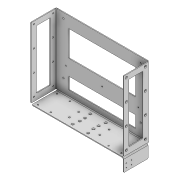
# Autodesk Inventor part: Display_Mount_A
Saved by Autodesk Inventor 2020 (Build 240168000, 168)
## iProperties
Created: 2021-12-05
Part Number: Display_Mount_A
Material: 一般
Document SubType Name: Sheet Metal
Designer: ken113
Density: 1 g/cm^3
Sheet Metal Rule: Default_mm
Appearance: 既定
Flat Pattern Width: 55.1572 cm
Flat Pattern Length: 37.0786 cm
Flat Pattern Area: 2045.15 cm^2
Sheet Metal Width: 551.572 mm
Sheet Metal Length: 370.786 mm
Sheet Metal Area: 204514.969 mm^2
Author: ken113
Autodesk Inventor part; units mm, degrees
ref_plane "YZ Plane" through (0, 0, 0) normal (1, 0, 0) x (0, 1, 0)
ref_plane "XZ Plane" through (0, 0, 0) normal (0, 1, 0) x (-1, 0, 0)
ref_plane "XY Plane" through (0, 0, 0) normal (0, 0, 1) x (1, 0, 0)
sketch "スケッチ1" plane through (0, 0, 0) normal (0, 0, 1) x (1, 0, 0)
  line L0 (175, -135) -> (-175, -135)
  line L1 (-175, -135) -> (-175, 135)
  line L2 (-175, 135) -> (175, 135)
  line L3 (175, 135) -> (175, -135)
  line L4 (175, -135) -> (-175, 135) construction
  line L5 (-175, -135) -> (175, 135) construction
  point P0 (0, 0)
  dimension "d0" = 270
  dimension "d1" = 350
  measures "d0" distance of L0.end L1.end
  measures "d1" distance of L1.end L2.end
extrude "プレート1" add sketch "スケッチ1" along normal blind 3
sketch "スケッチ2" plane through (175, -138, 6) normal (0, -1, 0) x (1, 0, 0)
  line L0 (-350, 0) -> (0, 0)
  line L1 (0, 0) -> (0, 94)
  line L2 (0, 94) -> (-350, 94)
  line L3 (-350, 94) -> (-350, 0)
  constraints: 6 end point, 1 horizontal, 1 perpendicular, 1 vertical
edge flange "フランジ1" height 100 angle 90 thickness 3 bend radius 3 thickness toward (0, -1, 0) relief straight relief width 3 relief depth 1.5 edges at (0, -135, 3) wall of the first edge with corners at (-175, -138, 6) (175, -138, 6) (175, -138, 100) (-175, -138, 100)
bend "曲げ1"
corner "コーナー1"
sketch "スケッチ3" plane through (0, 0, 3) normal (0, 0, 1) x (1, 0, 0)
  line L0 (150, -85) -> (-150, -85)
  line L1 (-150, -85) -> (-150, 115)
  line L2 (-150, 115) -> (150, 115)
  line L3 (150, 115) -> (150, -85)
  line L4 (150, -85) -> (-150, 115) construction
  line L5 (-150, -85) -> (150, 115) construction
  line L6 (175, -135) -> (-175, -135) projected
  point P0 (0, 0)
  point P1 (0, 15)
  dimension "d13" = 300
  dimension "d14" = 200
  dimension "d15" = 50
  constraints: 12 end point, 2 midpoint, 2 parallel, 1 horizontal, 1 perpendicular
  measures "d13" distance of L0.start L0.end
  measures "d14" distance of L0.end L1.end
  measures "d15" distance between parallel lines of L0 L6
hole "穴1" at (-150, 115, 3) at (-150, -85, 3) at (150, -85, 3) at (150, 115, 3) direction (0, 0, -1) diameter 6.2 depth 3 tip angle 118
sketch "スケッチ4" plane through (0, 0, 3) normal (0, 0, 1) x (1, 0, 0)
  line L0 (130, -8.8) -> (-130, -8.8)
  line L1 (-130, -8.8) -> (-130, 91.2)
  line L2 (-130, 91.2) -> (130, 91.2)
  line L3 (130, 91.2) -> (130, -8.8)
  line L4 (130, -8.8) -> (-130, 91.2) construction
  line L5 (-130, -8.8) -> (130, 91.2) construction
  circle A0 centre (-150, 115) radius 3.1 projected
  point P0 (0, 0)
  point P1 (0, 41.2)
  point P2 (0, 41.2)
  dimension "d23" = 100
  dimension "d24" = 23.8
  dimension "d25" = 260
  constraints: 12 end point, 3 midpoint, 2 parallel, 1 horizontal, 1 perpendicular, 1 vertical alignment
  measures "d23" distance of L2.end L0.start
  measures "d24" distance from line of L2 A0.centre
  measures "d25" distance of L1.end L2.end
extrude "押し出し1" cut sketch "スケッチ4" against normal through all contours L0 L1 L2 L3
fillet "フィレット1" radius 2 4 edges at (130, -8.8, 1.5) (130, 91.2, 1.5) (-130, 91.2, 1.5) (-130, -8.8, 1.5)
sketch "スケッチ5" plane through (-175, -138, 100) normal (0, 1, 0) x (1, 0, 0)
  line L0 (350, 94) -> (0, 94) projected
  line L1 (0, 0) -> (0, 94) projected
  line L2 (0, 0) -> (350, 0) projected
  line L3 (350, 0) -> (350, 94) projected
  line L4 (145, 13) -> (205, 13)
  line L5 (205, 13) -> (205, 81)
  line L6 (205, 81) -> (145, 81)
  line L7 (145, 81) -> (145, 13)
  line L8 (145, 13) -> (205, 81) construction
  line L9 (205, 13) -> (145, 81) construction
  line L10 (148.5, 37) -> (201.5, 37)
  line L11 (201.5, 37) -> (201.5, 57)
  line L12 (201.5, 57) -> (148.5, 57)
  line L13 (148.5, 57) -> (148.5, 37)
  line L14 (148.5, 37) -> (201.5, 57) construction
  line L15 (201.5, 37) -> (148.5, 57) construction
  point P0 (175, 100)
  point P1 (175, 47)
  point P2 (175, 0)
  point P3 (175, 47)
  point P4 (0, 47)
  point P5 (175, 47)
  dimension "d29" = 60
  dimension "d30" = 68
  dimension "d31" = 53
  dimension "d32" = 20
  constraints: 24 end point, 8 midpoint, 4 parallel, 2 horizontal, 2 perpendicular, 1 horizontal alignment, 1 vertical alignment
  measures "d29" distance of L6.end L5.end
  measures "d30" distance of L5.end L4.end
  measures "d31" distance of L12.end L11.end
  measures "d32" distance of L11.end L10.end
hole "穴2" at (-30, -138, 19) at (-26.5, -138, 43) at (-26.5, -138, 63) at (26.5, -138, 63) at (26.5, -138, 43) at (30, -138, 19) at (30, -138, 87) at (-30, -138, 87) direction (0, -1, 0) diameter 5.3 depth 3 tip angle 118 countersink diameter 10 countersink angle 90
sketch "スケッチ6" plane through (178, 135, 6) normal (1, 0, 0) x (0, 1, 0)
  line L0 (-270, 0) -> (0, 0)
  line L1 (0, 0) -> (0, 94)
  line L2 (0, 94) -> (-270, 94)
  line L3 (-270, 94) -> (-270, 0)
  constraints: 6 end point, 1 horizontal, 1 perpendicular, 1 vertical
edge flange "フランジ2" height 100 angle 90 thickness 3 bend radius 3 thickness toward (1, 0, 0) relief straight relief width 3 relief depth 1.5 corner gap 3 corner form 0 edges at (175, 0, 3) (-175, 0, 3) wall of the first edge with corners at (178, -135, 6) (178, 135, 6) (178, 135, 100) (178, -135, 100)
bend "曲げ2"
corner "コーナー2"
fillet "フィレット2" radius 2 5 edges at (-179.5, 135, 100) (-179.5, -135, 100) (-175, -139.5, 100) (179.5, -135, 100) (179.5, 135, 100)
sketch "スケッチ7" plane through (181, -135, 6) normal (1, 0, 0) x (0, 0, -1)
  arc A0 (-94, 268) -> (-92, 270) centre (-92, 268) ccw projected
  line L0 (-94, 2) -> (-94, 268) projected
  arc A1 (-92, 0) -> (-94, 2) centre (-92, 2) ccw projected
  line L1 (0, 0) -> (-92, 0) projected
  line L2 (0, 0) -> (0, 270) projected
  line L3 (-92, 270) -> (0, 270)
  line L4 (-10, 260) -> (-10, 16)
  line L5 (-10, 16) -> (-84, 16)
  line L6 (-84, 16) -> (-84, 260)
  line L7 (-84, 260) -> (-10, 260)
  line L8 (-84, 97.3333) -> (-10, 97.3333)
  line L9 (-10, 97.3333) -> (-10, 178.6667)
  line L10 (-10, 178.6667) -> (-84, 178.6667)
  line L11 (-84, 178.6667) -> (-84, 97.3333)
  point P0 (6, 135)
  dimension "d51" = 10
  dimension "d52" = 244
  dimension "d53" = 81.3333
  dimension "d54" = 81.3333
  dimension "d75" = 10
  dimension "d76" = 16
  dimension "d77" = 10
  constraints: 18 end point, 2 centre point, 2 parallel, 2 perpendicular, 2 point on line, 1 horizontal
  measures "d51" distance between parallel lines of L2 L4
  measures "d52" distance of L5.end L6.end
  measures "d53" distance between parallel lines of L7 L10
  measures "d54" distance between parallel lines of L10 L8
  measures "d75" distance between parallel lines of L6 L0
  measures "d76" distance between parallel lines of L5 L1
  measures "d77" distance between parallel lines of L3 L7
hole "穴3" at (181, 125, 90) at (181, 125, 16) at (181, 43.6667, 16) at (181, 43.6667, 90) at (181, -37.6667, 16) at (181, -37.6667, 90) at (181, -119, 90) at (181, -119, 16) direction (-1, 0, 0) diameter 5.3 depth 3 tip angle 118 countersink diameter 10 countersink angle 90
mirror "ミラー1" about plane through (0, 0, 0) normal (1, 0, 0) of "穴3"
sketch "スケッチ9" plane through (-175, -141, 6) normal (0, -1, 0) x (1, 0, 0)
  line L0 (2, 94) -> (350, 94) projected
  arc A0 (2, 94) -> (0, 92) centre (2, 92) ccw projected
  line L1 (0, 0) -> (0, 92) projected
  line L2 (0, 0) -> (350, 0) projected
  line L3 (350, 94) -> (350, 0) projected
  circle A1 centre (205, 81) radius 2.65 projected
  circle A2 centre (201.5, 37) radius 2.65 projected
  circle A3 centre (148.5, 57) radius 2.65 projected
  circle A4 centre (145, 13) radius 2.65 projected
  circle A5 centre (148.5, 37) radius 2.65 projected
  circle A6 centre (201.5, 57) radius 2.65 projected
  circle A7 centre (205, 13) radius 2.65 projected
  circle A8 centre (145, 81) radius 2.65 projected
  line L4 (13, 84) -> (63, 84)
  line L5 (63, 84) -> (63, 10)
  line L6 (63, 10) -> (13, 10)
  line L7 (13, 10) -> (13, 84)
  line L8 (287, 84) -> (337, 84)
  line L9 (337, 84) -> (337, 10)
  line L10 (337, 10) -> (287, 10)
  line L11 (287, 10) -> (287, 84)
  point P0 (175, -6)
  dimension "d62" = 13
  dimension "d63" = 10
  dimension "d64" = 10
  dimension "d65" = 13
  dimension "d66" = 50
  dimension "d67" = 50
  constraints: 16 end point, 4 parallel, 2 horizontal, 2 perpendicular, 2 point on line
  measures "d62" distance between parallel lines of L7 L1
  measures "d63" distance between parallel lines of L0 L4
  measures "d64" distance between parallel lines of L6 L2
  measures "d65" distance between parallel lines of L3 L9
  measures "d66" distance of L4.start L4.end
  measures "d67" distance of L8.start L8.end
hole "穴4" at (-162, -141, 16) at (-162, -141, 90) at (-112, -141, 90) at (-112, -141, 16) at (112, -141, 16) at (162, -141, 16) at (162, -141, 90) at (112, -141, 90) direction (0, 1, 0) diameter 5.2 depth 3 tip angle 118 countersink diameter 10 countersink angle 90
sketch "スケッチ10" plane through (-181, -135, 6) normal (-1, 0, 0) x (0, 0, 1)
  line L0 (20, 250) -> (74, 250)
  line L1 (74, 250) -> (74, 23)
  line L2 (74, 23) -> (20, 23)
  line L3 (20, 23) -> (20, 250)
  line L4 (0, 270) -> (92, 270) projected
  line L5 (94, 268) -> (94, 2) projected
  line L6 (0, 270) -> (0, 0) projected
  line L7 (92, 0) -> (0, 0) projected
  point P0 (-6, 135)
  dimension "d78" = 20
  dimension "d79" = 20
  dimension "d80" = 20
  dimension "d81" = 23
  constraints: 8 end point, 2 parallel, 1 horizontal, 1 perpendicular
  measures "d78" distance between parallel lines of L4 L0
  measures "d79" distance between parallel lines of L5 L1
  measures "d80" distance between parallel lines of L6 L3
  measures "d81" distance between parallel lines of L2 L7
extrude "押し出し2" cut sketch "スケッチ10" against normal through all
fillet "フィレット3" radius 2 8 edges at (-179.5, -112, 26) (-179.5, -112, 80) (-179.5, 115, 80) (-179.5, 115, 26) (179.5, 115, 26) (179.5, 115, 80) (179.5, -112, 80) (179.5, -112, 26)
sketch "スケッチ11" plane through (0, 0, 3) normal (0, 0, 1) x (1, 0, 0)
  line L0 (-128, 91.2) -> (128, 91.2) projected
  arc A0 (130, 89.2) -> (128, 91.2) centre (128, 89.2) ccw projected
  line L1 (130, 89.2) -> (130, -6.8) projected
  arc A1 (128, -8.8) -> (130, -6.8) centre (128, -6.8) ccw projected
  line L2 (128, -8.8) -> (-128, -8.8) projected
  arc A2 (-130, -6.8) -> (-128, -8.8) centre (-128, -6.8) ccw projected
  line L3 (-130, -6.8) -> (-130, 89.2) projected
  arc A3 (-128, 91.2) -> (-130, 89.2) centre (-128, 89.2) ccw projected
  circle A4 centre (150, -85) radius 3.1 projected
  circle A5 centre (-150, 115) radius 3.1 projected
  circle A6 centre (-150, -85) radius 3.1 projected
  circle A7 centre (150, 115) radius 3.1 projected
  line L4 (-175, -135) -> (-175, 135) projected
  line L5 (175, -135) -> (-175, -135) projected
  line L6 (175, 135) -> (175, -135) projected
  line L7 (-175, 135) -> (175, 135) projected
  point P0 (0, 0)
  point P1 (-140, -38.8)
  point P2 (0, -38.8)
  point P3 (140, -38.8)
  dimension "d87" = 140
  dimension "d92" = 30
  constraints: 1 horizontal, 1 vertical alignment, 2 other
  measures "d87" distance of point (-140, -38.8) point (0, -38.8)
  measures "d92" distance from line of point (-140, -38.8) L2
hole "穴5" at (-140, -38.8, 3) at (0, -38.8, 3) at (140, -38.8, 3) direction (0, 0, -1) diameter 4.2 end through all
sketch "スケッチ12" plane through (0, 0, 0) normal (0, 0, -1) x (-1, 0, 0)
  circle A0 centre (0, -38.8) radius 2.1 projected
  circle A1 centre (140, -38.8) radius 2.1 projected
  circle A2 centre (-140, -38.8) radius 2.1 projected
  line L0 (-128, 91.2) -> (128, 91.2) projected
  arc A3 (130, 89.2) -> (128, 91.2) centre (128, 89.2) ccw projected
  line L1 (130, 89.2) -> (130, -6.8) projected
  arc A4 (128, -8.8) -> (130, -6.8) centre (128, -6.8) ccw projected
  line L2 (128, -8.8) -> (-128, -8.8) projected
  arc A5 (-130, -6.8) -> (-128, -8.8) centre (-128, -6.8) ccw projected
  line L3 (-130, -6.8) -> (-130, 89.2) projected
  arc A6 (-128, 91.2) -> (-130, 89.2) centre (-128, 89.2) ccw projected
  circle A7 centre (-150, -85) radius 3.1 projected
  circle A8 centre (150, 115) radius 3.1 projected
  circle A9 centre (150, -85) radius 3.1 projected
  circle A10 centre (-150, 115) radius 3.1 projected
  line L4 (-175, -135) -> (175, -135) projected
  line L5 (175, -135) -> (175, 135) projected
  line L6 (175, 135) -> (-175, 135) projected
  line L7 (-175, 135) -> (-175, -135) projected
  point P0 (0, 0)
hole "穴6" at (140, -38.8, 0) at (0, -38.8, 0) at (-140, -38.8, 0) direction (0, 0, 1) diameter 4.3 end through all countersink diameter 8 countersink angle 90
sketch "スケッチ13" plane through (0, 0, 3) normal (0, 0, 1) x (1, 0, 0)
  circle A0 centre (0, -38.8) radius 2.15 projected
  circle A1 centre (-140, -38.8) radius 2.15 projected
  circle A2 centre (140, -38.8) radius 2.15 projected
  line L0 (-128, 91.2) -> (128, 91.2) projected
  arc A3 (130, 89.2) -> (128, 91.2) centre (128, 89.2) ccw projected
  line L1 (130, 89.2) -> (130, -6.8) projected
  arc A4 (128, -8.8) -> (130, -6.8) centre (128, -6.8) ccw projected
  line L2 (128, -8.8) -> (-128, -8.8) projected
  arc A5 (-130, -6.8) -> (-128, -8.8) centre (-128, -6.8) ccw projected
  line L3 (-130, -6.8) -> (-130, 89.2) projected
  arc A6 (-128, 91.2) -> (-130, 89.2) centre (-128, 89.2) ccw projected
  circle A7 centre (150, -85) radius 3.1 projected
  circle A8 centre (-150, 115) radius 3.1 projected
  circle A9 centre (-150, -85) radius 3.1 projected
  circle A10 centre (150, 115) radius 3.1 projected
  line L4 (-175, -135) -> (-175, 135) projected
  line L5 (175, -135) -> (-175, -135) projected
  line L6 (175, 135) -> (175, -135) projected
  line L7 (-175, 135) -> (175, 135) projected
  line L8 (-129.4142, -68.8) -> (130, -68.8)
  line L9 (130, -68.8) -> (130, -115)
  line L10 (130, -115) -> (-129.4142, -115)
  line L11 (-129.4142, -115) -> (-129.4142, -68.8)
  point P0 (0, 0)
  dimension "d107" = 30
  dimension "d108" = 20
  constraints: 8 end point, 2 parallel, 1 horizontal, 1 perpendicular, 1 vertical alignment
  measures "d107" distance from line of A0.centre L8
  measures "d108" distance between parallel lines of L10 L5
extrude "押し出し3" cut sketch "スケッチ13" against normal blind 10 contours L8 L9 L10 L11
fillet "フィレット4" radius 2 4 edges at (-129.4142, -68.8, 1.5) (-129.4142, -115, 1.5) (130, -115, 1.5) (130, -68.8, 1.5)
sketch "スケッチ14" plane through (-175, -138, 6) normal (0, 1, 0) x (1, 0, 0)
  circle A0 centre (337, -84) radius 2.6 projected
  circle A1 centre (287, -10) radius 2.6 projected
  circle A2 centre (63, -84) radius 2.6 projected
  circle A3 centre (13, -10) radius 2.6 projected
  circle A4 centre (13, -84) radius 2.6 projected
  circle A5 centre (63, -10) radius 2.6 projected
  circle A6 centre (337, -10) radius 2.6 projected
  circle A7 centre (287, -84) radius 2.6 projected
  circle A8 centre (205, -81) radius 5 projected
  circle A9 centre (201.5, -37) radius 5 projected
  circle A10 centre (148.5, -57) radius 5 projected
  circle A11 centre (145, -13) radius 5 projected
  circle A12 centre (148.5, -37) radius 5 projected
  circle A13 centre (201.5, -57) radius 5 projected
  circle A14 centre (205, -13) radius 5 projected
  circle A15 centre (145, -81) radius 5 projected
  line L0 (350, -94) -> (350, 0) projected
  line L1 (350, 0) -> (0, 0) projected
  line L2 (0, -92) -> (0, 0) projected
  arc A16 (0, -92) -> (2, -94) centre (2, -92) ccw projected
  line L3 (2, -94) -> (350, -94) projected
  circle A17 centre (148.5, -57) radius 2.65 projected
  line L4 (148.5, -57) -> (201.5, -57)
  line L5 (201.5, -57) -> (201.5, -37)
  line L6 (201.5, -37) -> (148.5, -37)
  line L7 (148.5, -37) -> (148.5, -57)
  line L8 (234, -65) -> (116, -65)
  line L9 (116, -65) -> (116, -29)
  line L10 (116, -29) -> (234, -29)
  line L11 (234, -29) -> (234, -65)
  line L12 (234, -65) -> (116, -29) construction
  line L13 (116, -65) -> (234, -29) construction
  point P0 (175, 6)
  point P1 (175, -47)
  point P2 (175, -37)
  point P3 (175, -47)
  point P4 (148.5, -47)
  point P5 (175, -47)
  dimension "d112" = 118
  dimension "d113" = 36
  constraints: 20 end point, 6 midpoint, 4 parallel, 2 horizontal, 2 perpendicular, 1 horizontal alignment, 1 vertical alignment
  measures "d112" distance of L9.end L10.end
  measures "d113" distance of L8.end L9.end
hole "穴7" at (-59, -138, 35) at (-59, -138, 71) at (59, -138, 71) at (59, -138, 35) direction (0, -1, 0) diameter 6.3 end through all
sketch "スケッチ15" plane through (178, -144, 100) normal (1, 0, 0) x (0, 1, 0)
  line L0 (0, -94) -> (0, 0)
  line L1 (0, 0) -> (-45, 0)
  line L2 (-45, 0) -> (-45, -94)
  line L3 (-45, -94) -> (0, -94)
  constraints: 6 end point, 1 horizontal, 1 perpendicular, 1 vertical
edge flange "フランジ3" height 51 angle 90 thickness 3 bend radius 3 thickness toward (1, 0, 0) relief straight relief width 3 relief depth 1.5 edges at (175, -141, 53) wall of the first edge with corners at (178, -144, 6) (178, -144, 100) (178, -189, 100) (178, -189, 6)
bend "曲げ3"
corner "コーナー3"
fillet "フィレット5" radius 2 2 edges at (179.5, -189, 100) (179.5, -189, 6)
sketch "スケッチ16" plane through (181, -144, 100) normal (1, 0, 0) x (0, 0, -1)
  line L0 (10, -33) -> (30, -33)
  line L1 (30, -33) -> (30, -18)
  line L2 (30, -18) -> (10, -18)
  line L3 (10, -18) -> (10, -33)
  line L4 (92, -45) -> (2, -45) projected
  line L5 (0, -43) -> (0, 0) projected
  point P0 (100, 144)
  point P1 (10, -25.5)
  dimension "d132" = 15
  dimension "d133" = 19.5
  dimension "d134" = 10
  dimension "d135" = 20
  constraints: 8 end point, 2 parallel, 1 horizontal, 1 midpoint, 1 perpendicular
  measures "d132" distance of L2.end L0.start
  measures "d133" distance from line of point (10, -25.5) L4
  measures "d134" distance between parallel lines of L3 L5
  measures "d135" distance of L0.start L0.end
hole "穴8" at (181, -162, 90) at (181, -177, 90) at (181, -162, 70) at (181, -177, 70) direction (-1, 0, 0) diameter 3.242 depth 11.8 tip angle 118 thread size "M4x0.7" class "6H" standard "ISO Metric profile"
equation "\"d21\" = Thickness"
equation "\"d38\" = Thickness"
equation "\"d53\" = 0.333333 * d52"
equation "\"d54\" = d53"
equation "\"d60\" = Thickness"
equation "\"d73\" = Thickness"
equation "\"d98\" = Thickness"
equation "\"d105\" = Thickness"
equation "\"d119\" = Thickness"
equation "\"d2\" = Thickness"
equation "\"d3\" = BendReliefWidth"
equation "\"d4\" = BendReliefDepth"
equation "\"d5\" = MinimumRemnant"
equation "\"d6\" = TransitionRadius"
equation "\"d9\" = BendRadius"
equation "\"d10\" = CornerReliefSize"
equation "\"d11\" = GapSize"
equation "\"d12\" = JacobiRadiusSize"
equation "\"d40\" = BendReliefWidth"
equation "\"d41\" = BendReliefDepth"
equation "\"d42\" = MinimumRemnant"
equation "\"d43\" = TransitionRadius"
equation "\"d46\" = BendRadius"
equation "\"d47\" = CornerReliefSize"
equation "\"d48\" = GapSize"
equation "\"d49\" = JacobiRadiusSize"
equation "\"d121\" = BendReliefWidth"
equation "\"d122\" = BendReliefDepth"
equation "\"d123\" = MinimumRemnant"
equation "\"d124\" = TransitionRadius"
equation "\"d127\" = BendRadius"
equation "\"d128\" = CornerReliefSize"
equation "\"d129\" = GapSize"
equation "\"d130\" = JacobiRadiusSize"
equation "\"BendRadius\" = Thickness"
equation "\"BendReliefWidth\" = Thickness"
equation "\"BendReliefDepth\" = 0.5 * Thickness"
equation "\"CornerReliefSize\" = 4 * Thickness"
equation "\"MinimumRemnant\" = 2 * Thickness"
equation "\"TransitionRadius\" = BendRadius"
equation "\"JacobiRadiusSize\" = BendRadius"
equation "\"GapSize\" = Thickness"
equation "\"Thickness\" = 3"
